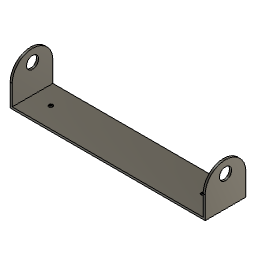
_Paper roll arm bracket.b6dafd9f-6d07-430f-9bc5-a98820684cc9 (Autodesk Fusion 360 design; units mm, degrees)
Autodesk Fusion 360 part; units mm, degrees
sketch "Sketch1" plane through (0, 0, 0) normal (0, 0, 1) x (1, 0, 0)
  line L0 (0, 0) -> (480, 0)
  line L1 (480, 0) -> (480, 100)
  line L2 (480, 100) -> (0, 100)
  line L3 (0, 100) -> (0, 0)
  dimension "d1" = 480
  dimension "d2" = 100
  constraint horizontal L0
  constraint vertical L1
  constraint horizontal L2
  constraint vertical L3
  constraint coincident L0.start L3.end
  measures "d1" distance of L0.start L0.end
  measures "d2" distance of L0.start L2.end
extrude "Extrude1" add sketch "Sketch1" along normal blind 5
sketch "Sketch2" plane through (0, 0, 5) normal (0, 0, 1) x (-1, 0, 0)
  line L0 (0, -100) -> (0, 0)
  line L1 (0, 0) -> (-480, 0)
  line L2 (-480, 0) -> (-480, -100)
  line L3 (-480, -100) -> (0, -100)
  line L4 (0, -100) -> (-5, -100)
  line L5 (-5, -100) -> (-5, 0)
  line L6 (-5, 0) -> (0, 0)
  line L7 (0, 0) -> (0, -100)
  line L8 (-480, -100) -> (-475, -100)
  line L9 (-475, -100) -> (-475, 0)
  line L10 (-475, 0) -> (-480, 0)
  line L11 (-480, 0) -> (-480, -100)
  dimension "d5" = 5
  dimension "d6" = 100
  dimension "d7" = 5
  dimension "d8" = 100
  constraint horizontal L4
  constraint vertical L5
  constraint horizontal L6
  constraint vertical L7
  constraint coincident L0.start L3.end
  constraint horizontal L8
  constraint vertical L9
  constraint horizontal L10
  constraint vertical L11
  constraint coincident L2.end L3.start
  measures "d5" distance of L0.start L4.end
  measures "d6" distance of L0.start L0.end
  measures "d7" distance of L2.end L8.end
  measures "d8" distance of L2.end L1.end
extrude "Extrude2" add sketch "Sketch2" along normal blind 100 contours L0 L1 L3 L4 L5 L6 L7 | L1 L2 L3 L8 L9 L10 L11
sketch "Sketch3" plane through (480, 0, 0) normal (1, 0, 0) x (0, 1, 0)
  line L0 (0, 0) -> (100, 0)
  line L1 (100, 0) -> (100, 105)
  line L2 (100, 105) -> (0, 105)
  line L3 (0, 105) -> (0, 0)
  circle A0 centre (50, 75) radius 15
  dimension "d11" = 30
  measures "d11" diameter of A0
extrude "Extrude3" cut sketch "Sketch3" against normal blind 500 contours A0
sketch "Sketch4" plane through (0, 0, 5) normal (0, 0, 1) x (-1, 0, 0)
  line L0 (-5, -100) -> (-5, 0)
  line L1 (-5, 0) -> (-475, 0)
  line L2 (-475, 0) -> (-475, -100)
  line L3 (-475, -100) -> (-5, -100)
  circle A0 centre (-50, -50) radius 5
  circle A1 centre (-425, -50) radius 5
  dimension "d14" = 10
  dimension "d15" = 10
  measures "d14" diameter of A0
  measures "d15" diameter of A1
extrude "Extrude4" cut sketch "Sketch4" against normal blind 2 contours A0 | A1
sketch "Sketch5" plane through (0, 0, 5) normal (0, 0, 1) x (-1, 0, 0)
  circle A0 centre (-425, -50) radius 5
  circle A1 centre (-50, -50) radius 5
  line L0 (-5, -100) -> (-5, 0)
  line L1 (-5, 0) -> (-475, 0)
  line L2 (-475, 0) -> (-475, -100)
  line L3 (-475, -100) -> (-5, -100)
  circle A2 centre (-50, -50) radius 3
  circle A3 centre (-425, -50) radius 3
  dimension "d18" = 6
  dimension "d19" = 6
  constraint concentric A1 A2
  constraint concentric A0 A3
  measures "d18" diameter of A2
  measures "d19" diameter of A3
extrude "Extrude5" cut sketch "Sketch5" against normal blind 6 contours A2 | A3
fillet "Fillet1" radius 50 4 edges at (477.5, 0, 105) (477.5, 100, 105) (2.5, 100, 105) (2.5, 0, 105)
